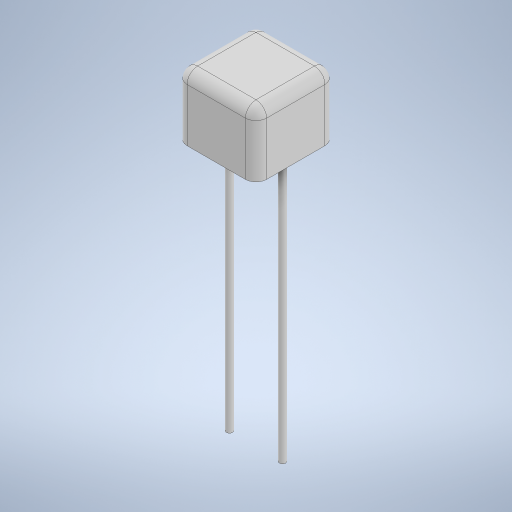
# Autodesk Inventor part: 54
Saved by Autodesk Inventor 2024 (Build 280153000, 153)
## iProperties
Created: 2023-12-01
Part Number: 54
Material: Generic
Document SubType Name: Sheet Metal
Designer: Shado
Density: 1 g/cm^3
Sheet Metal Rule: Default
Appearance: Default
Author: Shado
Autodesk Inventor part; units mm, degrees
ref_plane "YZ Plane" through (0, 0, 0) normal (1, 0, 0) x (0, 1, 0)
ref_plane "XZ Plane" through (0, 0, 0) normal (0, 1, 0) x (-1, 0, 0)
ref_plane "XY Plane" through (0, 0, 0) normal (0, 0, 1) x (1, 0, 0)
sketch "Sketch2" plane through (0, 0, 0) normal (1, 0, 0) x (0, 1, 0)
  line L0 (0, 0) -> (6, 0)
  line L1 (6, 0) -> (6, 3.75)
  line L2 (6, 3.75) -> (0, 3.75)
  line L3 (0, 3.75) -> (0, 0)
  line L4 (6, 0) -> (0, 0)
  line L5 (0, 0) -> (0, -3.75)
  line L6 (0, -3.75) -> (6, -3.75)
  line L7 (6, -3.75) -> (6, 0)
  dimension "d3" = 6
  dimension "d4" = 3.75
  dimension "d5" = 3.75
  constraints: 16 end point, 4 parallel, 2 horizontal, 2 perpendicular
  measures "d3" distance of L2.end L1.end
  measures "d4" distance of L1.end L0.end
  measures "d5" distance of L5.end L4.end
extrude "Extrusion1" add sketch "Sketch2" along normal blind 3.75 and the other way blind 3.75
fillet "Fillet1" radius 1 4 edges at (0, 6, 3.75) (3.75, 6, 0) (-3.75, 6, 0) (0, 6, -3.75)
fillet "Fillet2" radius 1 8 edges at (3.4571, 5.7071, 3.4571) (3.75, 2.5, 3.75) (-3.4571, 5.7071, 3.4571) (-3.75, 2.5, 3.75) (-3.4571, 5.7071, -3.4571) (-3.75, 2.5, -3.75) (3.4571, 5.7071, -3.4571) (3.75, 2.5, -3.75)
sketch "Sketch3" plane through (-2.75, 0, 3.75) normal (0, -1, 0) x (1, 0, 0)
  line L0 (0, 0) -> (5.5, 0) projected
  line L1 (2.75, 0) -> (2.75, -7.5)
  line L2 (5.5, -7.5) -> (0, -7.5) projected
  circle A0 centre (5.25, -3.75) radius 0.3
  circle A1 centre (0.25, -3.75) radius 0.3
  point P0 (2.75, -3.75)
  dimension "d13" = 0.6
  dimension "d14" = 0.6
  constraints: 2 centre point, 2 end point, 2 midpoint
  measures "d13" diameter of A0
  measures "d14" diameter of A1
extrude "Extrusion2" add sketch "Sketch3" along normal blind 25
fillet "Fillet3" radius 0.2 2 edges at (2.2, 0, 0) (-2.8, 0, 0) inverted yes
equation "\"BendRadius\" = Thickness"
equation "\"BendReliefWidth\" = Thickness"
equation "\"BendReliefDepth\" = 0.5 * Thickness"
equation "\"CornerReliefSize\" = 4 * Thickness"
equation "\"MinimumRemnant\" = 2 * Thickness"
equation "\"TransitionRadius\" = BendRadius"
equation "\"JacobiRadiusSize\" = BendRadius"
equation "\"GapSize\" = Thickness"
equation "\"Thickness\" = 3.048"
body "Solid1"
